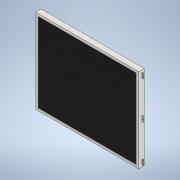
# Autodesk Inventor part: skærm
Saved by Autodesk Inventor 2022 (Build 260153000, 153)
## iProperties
Created: 2023-08-31
Part Number: skærm
Material: Generic
Document SubType Name: Modeling
Designer: THK
Density: 1 g/cm^3
Appearance: Steel
Author: THK
Autodesk Inventor part; units mm, degrees
ref_plane "YZ Plane" through (0, 0, 0) normal (1, 0, 0) x (0, 1, 0)
ref_plane "XZ Plane" through (0, 0, 0) normal (0, 1, 0) x (-1, 0, 0)
ref_plane "XY Plane" through (0, 0, 0) normal (0, 0, 1) x (1, 0, 0)
sketch "Sketch1" plane through (0, 0, 0) normal (0, 0, 1) x (1, 0, 0)
  line L0 (-199, 163) -> (199, 163)
  line L1 (199, 163) -> (199, -163)
  line L2 (199, -163) -> (-199, -163)
  line L3 (-199, -163) -> (-199, 163)
  line L4 (-199, 163) -> (199, -163) construction
  line L5 (199, 163) -> (-199, -163) construction
  point P0 (0, 0)
  dimension "d0" = 398
  dimension "d1" = 326
  constraints: 12 end point, 2 midpoint, 2 parallel, 1 horizontal, 1 perpendicular
  measures "d0" distance of L1.end L2.end
  measures "d1" distance of L0.end L1.end
extrude "Extrusion1" add sketch "Sketch1" against normal blind 21
ref_plane "Work Plane1" through (0, 0, -12) normal (0, 0, 1) x (1, 0, 0)
sketch "Sketch2" plane through (0, 0, -12) normal (0, 0, 1) x (1, 0, 0)
  line L0 (-206, 163) -> (206, 163) construction
  line L1 (206, -170) -> (-206, -170) construction
  line L2 (-206, -170) -> (-206, 163) construction
  line L3 (-206, 163) -> (206, -170) construction
  line L4 (206, 163) -> (-206, -170) construction
  line L5 (-199, -163) -> (199, -163) construction
  line L6 (-199, 163) -> (-199, -163) construction
  line L7 (199, 163) -> (-199, 163) construction
  line L8 (-199, -163) -> (-199, 163) projected
  line L9 (199, 10.5) -> (206, 10.5)
  line L10 (206, 10.5) -> (206, -10.5)
  line L11 (206, -10.5) -> (199, -10.5)
  line L12 (199, -10.5) -> (199, 10.5)
  line L13 (199, 10.5) -> (206, -10.5) construction
  line L14 (206, 10.5) -> (199, -10.5) construction
  line L15 (206, -134.9) -> (199, -134.9)
  line L16 (199, -134.9) -> (199, -154.9)
  line L17 (199, -154.9) -> (206, -154.9)
  line L18 (206, -154.9) -> (206, -134.9)
  line L19 (199, -163) -> (-199, -163) projected
  line L20 (-8, -163) -> (8, -163)
  line L21 (8, -163) -> (8, -170)
  line L22 (8, -170) -> (-8, -170)
  line L23 (-8, -170) -> (-8, -163)
  line L24 (-139, -163) -> (-119, -163)
  line L25 (-119, -163) -> (-119, -170)
  line L26 (-119, -170) -> (-139, -170)
  line L27 (-139, -170) -> (-139, -163)
  line L28 (119, -163) -> (139, -163)
  line L29 (139, -163) -> (139, -170)
  line L30 (139, -170) -> (119, -170)
  line L31 (119, -170) -> (119, -163)
  line L32 (206, 163) -> (206, -170) construction
  line L33 (199, -163) -> (199, 163) projected
  line L34 (-288.4, 0) -> (288.4, 0) projected
  line L35 (0, 229.6) -> (0, -236.6) projected
  line L36 (206, 134.9) -> (199, 134.9)
  line L37 (199, 134.9) -> (199, 154.9)
  line L38 (199, 154.9) -> (206, 154.9)
  line L39 (206, 154.9) -> (206, 134.9)
  line L40 (-199, 10.5) -> (-206, 10.5)
  line L41 (-206, 10.5) -> (-206, -10.5)
  line L42 (-206, -10.5) -> (-199, -10.5)
  line L43 (-199, -10.5) -> (-199, 10.5)
  line L44 (-199, 10.5) -> (-206, -10.5) construction
  line L45 (-206, 10.5) -> (-199, -10.5) construction
  line L46 (-206, -134.9) -> (-199, -134.9)
  line L47 (-199, -134.9) -> (-199, -154.9)
  line L48 (-199, -154.9) -> (-206, -154.9)
  line L49 (-206, -154.9) -> (-206, -134.9)
  line L50 (-199, 134.9) -> (-199, 154.9)
  line L51 (-206, 134.9) -> (-199, 134.9)
  line L52 (-206, 154.9) -> (-206, 134.9)
  line L53 (-199, 154.9) -> (-206, 154.9)
  point P0 (0, 0)
  point P1 (0, -3.5)
  point P2 (202.5, 0)
  point P3 (202.5, 0)
  point P4 (-202.5, 0)
  point P5 (-202.5, 0)
  point P6 (0, -170)
  dimension "d6" = 7
  dimension "d7" = 7
  dimension "d8" = 0
  dimension "d9" = 21
  dimension "d10" = 20
  dimension "d11" = 124.4
  dimension "d12" = 7
  dimension "d13" = 16
  dimension "d14" = 111
  dimension "d15" = 20
  dimension "d16" = 111
  dimension "d17" = 20
  constraints: 92 end point, 18 symmetric about line, 11 parallel, 10 point on line, 8 midpoint, 6 horizontal, 5 perpendicular, 1 horizontal alignment, 1 vertical, 1 vertical alignment
  measures "d6" distance between parallel lines of L5 L1
  measures "d7" distance between parallel lines of L6 L2
  measures "d8" distance between parallel lines of L7 L0
  measures "d9" distance between parallel lines of L11 L9
  measures "d10" distance between parallel lines of L17 L15
  measures "d11" distance between parallel lines of L15 L11
  measures "d12" distance between parallel lines of L33 L32
  measures "d13" distance between parallel lines of L21 L23
  measures "d14" distance between parallel lines of L31 L21
  measures "d15" distance between parallel lines of L29 L31
  measures "d16" distance between parallel lines of L25 L23
  measures "d17" distance between parallel lines of L25 L27
extrude "Extrusion2" add sketch "Sketch2" against normal blind 1 contours L48 L49 L46 L8 | L19 L25 L26 L27 | L42 L41 L34 L8 | L19 L35 L22 L23 | L34 L41 L40 L8 | L19 L21 L22 L35 | L34 L10 L11 L12 | L12 L9 L10 L34 | L19 L29 L30 L31 | L15 L18 L17 L16 | L51 L52 L53 L8 | L33 L38 L39 L36
sketch "Sketch3" plane through (0, 0, -12) normal (0, 0, 1) x (1, 0, 0)
  line L0 (-119, -170) -> (-119, -163) projected
  line L1 (8, -170) -> (8, -163) projected
  line L2 (119, -163) -> (119, -170) projected
  point P0 (0, 0)
  point P1 (-202.5, 0)
  point P2 (202.5, 0)
  point P3 (129, -166.5)
  point P4 (0, -166.5)
  point P5 (-129, -166.5)
  point P6 (-119, -166.5)
  point P7 (8, -166.5)
  point P8 (119, -166.5)
  constraints: 3 horizontal alignment, 3 midpoint
hole "Hole1" at (-202.5, 0, -12) at (202.5, 0, -12) at (129, -166.5, -12) at (0, -166.5, -12) at (-129, -166.5, -12) direction (0, 0, -1) diameter 4 end through all
sketch "Sketch4" plane through (0, 0, -12) normal (0, 0, 1) x (1, 0, 0)
  line L0 (206, -134.9) -> (199, -134.9) projected
  point P0 (0, 0)
  point P1 (202.5, -139.9)
  dimension "d27" = 5
  measures "d27" distance from line of point (202.5, -139.9) L0
hole "Hole2" at (202.5, -139.9, -12) direction (0, 0, -1) diameter 4 end through all
sketch "Sketch5" plane through (0, 0, -12) normal (0, 0, 1) x (1, 0, 0)
  line L0 (199, -154.9) -> (206, -154.9) projected
  point P0 (0, 0)
  point P1 (202.5, -148.4)
  point P2 (202.5, -154.9)
  dimension "d35" = 6.5
  constraints: 1 midpoint, 1 vertical alignment
  measures "d35" distance from line of L0 point (202.5, -148.4)
hole "Hole3" at (202.5, -148.4, -12) direction (0, 0, -1) diameter 6 end through all
mirror "Mirror1" about plane through (0, 0, 0) normal (0, 1, 0) of "Hole2", "Hole3"
mirror "Mirror2" about plane through (0, 0, 0) normal (1, 0, 0) of "Hole2", "Hole3", "Mirror1"
sketch "Sketch6" plane through (0, 0, 0) normal (0, 0, 1) x (1, 0, 0)
  line L0 (-199, -163) -> (199, -163) projected
  line L1 (199, -163) -> (199, 163) projected
  line L2 (199, 163) -> (-199, 163) projected
  line L3 (-199, 163) -> (-199, -163) projected
  line L4 (-189.5, 153.5) -> (189.5, 153.5)
  line L5 (189.5, 153.5) -> (189.5, -153.5)
  line L6 (189.5, -153.5) -> (-189.5, -153.5)
  line L7 (-189.5, -153.5) -> (-189.5, 153.5)
  point P0 (0, 0)
  dimension "d43" = 9.5
  constraints: 8 end point, 3 other
  measures "d43" distance between parallel lines of L2 L4
extrude "Extrusion3" cut sketch "Sketch6" against normal blind 1 contours L4 L5 L6 L7
body "Solid1"
